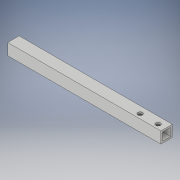
# Autodesk Inventor part: arm
Saved by Autodesk Inventor 2019 (Build 230136000, 136)
## iProperties
Created: 2019-02-02
Part Number: arm
Material: Generic
Document SubType Name: Modeling
Designer: suchanek
Density: 1 g/cm^3
Appearance: Default
Author: suchanek
Autodesk Inventor part; units mm, degrees
ref_plane "YZ Plane" through (0, 0, 0) normal (1, 0, 0) x (0, 1, 0)
ref_plane "XZ Plane" through (0, 0, 0) normal (0, 1, 0) x (-1, 0, 0)
ref_plane "XY Plane" through (0, 0, 0) normal (0, 0, 1) x (1, 0, 0)
sketch "Sketch1" plane through (0, 0, 0) normal (1, 0, 0) x (0, 1, 0)
  line L0 (-6.35, 6.35) -> (6.35, 6.35)
  line L1 (6.35, 6.35) -> (6.35, -6.35)
  line L2 (6.35, -6.35) -> (-6.35, -6.35)
  line L3 (-6.35, -6.35) -> (-6.35, 6.35)
  line L4 (-6.35, 6.35) -> (6.35, -6.35) construction
  line L5 (6.35, 6.35) -> (-6.35, -6.35) construction
  line L6 (-4.35, 4.35) -> (4.35, 4.35)
  line L7 (4.35, 4.35) -> (4.35, -4.35)
  line L8 (4.35, -4.35) -> (-4.35, -4.35)
  line L9 (-4.35, -4.35) -> (-4.35, 4.35)
  line L10 (-4.35, 4.35) -> (4.35, -4.35) construction
  line L11 (4.35, 4.35) -> (-4.35, -4.35) construction
  point P0 (0, 0)
  dimension "d0" = 12.7
  dimension "d1" = 12.7
  dimension "d13" = 2
  dimension "d14" = 2
  constraints: 24 end point, 4 midpoint, 4 parallel, 2 horizontal, 2 perpendicular
  measures "d0" distance of L1.end L2.end
  measures "d1" distance of L0.end L1.end
  measures "d13" distance between parallel lines of L2 L8
  measures "d14" distance between parallel lines of L1 L7
extrude "Extrusion1" add sketch "Sketch1" along normal blind 170
sketch "Sketch2" plane through (0, 6.35, 6.35) normal (0, 1, 0) x (1, 0, 0)
  circle A0 centre (162, 5) radius 2.6
  line L0 (170, 12.7) -> (170, 0) projected
  circle A1 centre (142, 5) radius 2.6
  line L1 (0, 0) -> (170, 0) projected
  point P0 (0, 6.35)
  dimension "d8" = 5.2
  dimension "d9" = 8
  dimension "d10" = 5.2
  dimension "d11" = 20
  dimension "d12" = 5
  constraints: 2 centre point, 1 horizontal alignment
  measures "d8" diameter of A0
  measures "d9" distance from line of L0 A0.centre
  measures "d10" diameter of A1
  measures "d11" distance of A0.centre A1.centre
  measures "d12" distance from line of L1 A0.centre
extrude "Extrusion2" cut sketch "Sketch2" against normal blind 10
equation "\"d1\" = d0"
equation "\"d14\" = d13"
body "Solid1"
